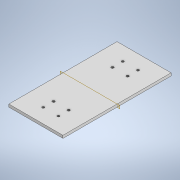
# Autodesk Inventor part: Aluminum_Heatsink_Base
Saved by Autodesk Inventor 2020 (Build 240168000, 168)
## iProperties
Created: 2019-11-19
Part Number: Aluminum_Heatsink_Base
Material: Generic
Document SubType Name: Modeling
Designer: kylew
Density: 1 g/cm^3
Appearance: Default
Author: kylew
Autodesk Inventor part; units mm, degrees
ref_plane "YZ Plane" through (0, 0, 0) normal (1, 0, 0) x (0, 1, 0)
ref_plane "XZ Plane" through (0, 0, 0) normal (0, 1, 0) x (-1, 0, 0)
sketch "Sketch1" plane through (0, 0, 0) normal (0, 1, 0) x (-1, 0, 0)
  line L0 (50, 100) -> (-50, 100)
  line L1 (-50, 100) -> (-50, -100)
  line L2 (-50, -100) -> (50, -100)
  line L3 (50, -100) -> (50, 100)
  line L4 (50, 100) -> (-50, -100) construction
  line L5 (-50, 100) -> (50, -100) construction
  point P0 (0, 0)
  dimension "d0" = 100
  dimension "d1" = 200
  constraints: 12 end point, 2 midpoint, 2 parallel, 1 horizontal, 1 perpendicular
  measures "d0" distance of L2.end L1.end
  measures "d1" distance of L1.end L0.end
extrude "Extrusion1" add sketch "Sketch1" along normal blind 5
sketch "Sketch2" plane through (0, 5, 0) normal (0, 1, 0) x (1, 0, 0)
  line L0 (-34.6, -58) -> (34.6, -58)
  line L1 (34.6, -58) -> (34.6, 58)
  line L2 (34.6, 58) -> (-34.6, 58)
  line L3 (-34.6, 58) -> (-34.6, -58)
  line L4 (-34.6, -58) -> (34.6, 58) construction
  line L5 (34.6, -58) -> (-34.6, 58) construction
  circle A0 centre (-12.9, 54.5) radius 2.5
  circle A1 centre (15.1, 54.5) radius 2.5
  line L6 (0, 0) -> (-70, 0) construction
  line L7 (0, 0) -> (70, 0) construction
  circle A2 centre (-12.9, -54.5) radius 2.5
  circle A3 centre (15.1, -54.5) radius 2.5
  dimension "d4" = 69.2
  dimension "d5" = 116
  dimension "d6" = 19.5
  dimension "d7" = 28
  dimension "d8" = 3.5
  dimension "d9" = 3.5
  dimension "d10" = 5
  dimension "d11" = 5
  dimension "d12" = 70
  dimension "d13" = 180
  constraints: 16 end point, 4 centre point, 3 horizontal, 2 midpoint, 2 parallel, 2 symmetric about line, 1 collinear, 1 perpendicular, 2 other
  measures "d4" distance of L2.end L1.end
  measures "d5" distance of L1.end L0.end
  measures "d6" distance from line of L1 A1.centre
  measures "d7" distance of A0.centre A1.centre
  measures "d8" distance from line of L2 A1.centre
  measures "d9" distance from line of L2 A0.centre
  measures "d10" diameter of A0
  measures "d11" diameter of A1
  measures "d12" distance of L6.start L6.end
  measures "d13" angle of L6 L7
hole "Hole1" at (-12.9, 5, 54.5) at (15.1, 5, 54.5) at (-12.9, 5, -54.5) at (15.1, 5, -54.5) direction (0, -1, 0) diameter 4.4587 end through all thread size "M5x0.5" class "6H" standard "ANSI Metric M Profile"
sketch "Sketch3" plane through (0, 5, 0) normal (0, 1, 0) x (1, 0, 0)
  line L0 (-34.6, -81) -> (34.6, -81)
  line L1 (34.6, -81) -> (34.6, 81)
  line L2 (34.6, 81) -> (-34.6, 81)
  line L3 (-34.6, 81) -> (-34.6, -81)
  line L4 (-34.6, -81) -> (34.6, 81) construction
  line L5 (34.6, -81) -> (-34.6, 81) construction
  point P0 (0, 0)
  point P1 (15.1, -73.5)
  point P2 (-12.9, -73.5)
  dimension "d21" = 69.2
  dimension "d22" = 162
  dimension "d23" = 7.5
  dimension "d24" = 7.5
  dimension "d25" = 28
  dimension "d26" = 19.5
  constraints: 12 end point, 2 midpoint, 2 parallel, 1 horizontal, 1 perpendicular
  measures "d21" distance of L2.end L1.end
  measures "d22" distance of L1.end L0.end
  measures "d23" distance from line of L0 point (15.1, -73.5)
  measures "d24" distance from line of L0 point (-12.9, -73.5)
  measures "d25" distance of point (15.1, -73.5) point (-12.9, -73.5)
  measures "d26" distance from line of L1 point (15.1, -73.5)
hole "Hole2" at (15.1, 5, 73.5) at (-12.9, 5, 73.5) direction (0, -1, 0) diameter 4.134 end through all thread size "M5x0.8" class "6H" standard "ANSI Metric M Profile"
mirror "Mirror2" about plane through (0, 0, 0) normal (0, 0, 1) of "Hole2"
body "Solid1"
